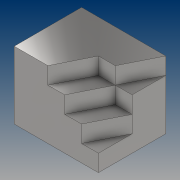
# Autodesk Inventor part: 23
Saved by Autodesk Inventor 2020.2 (Build 242310000, 310)
## iProperties
Created: 2020-09-17
Part Number: 23
Material: 鋼、碳鋼
Document SubType Name: Modeling
Designer: user
Density: 7.85 g/cm^3
Appearance: 半拋光
Mass: 549.5 g
Surface Area: 108.944 cm^2
Volume: 70 cm^3
Author: user
Autodesk Inventor part; units mm, degrees
ref_plane "YZ Plane" through (0, 0, 0) normal (1, 0, 0) x (0, 1, 0)
ref_plane "XZ Plane" through (0, 0, 0) normal (0, 1, 0) x (-1, 0, 0)
ref_plane "XY Plane" through (0, 0, 0) normal (0, 0, 1) x (1, 0, 0)
sketch "草圖1" plane through (0, 0, 0) normal (0, 1, 0) x (-1, 0, 0)
  line L0 (-25, 20) -> (25, 20)
  line L1 (25, 20) -> (25, -20)
  line L2 (25, -20) -> (-25, -20)
  line L3 (-25, -20) -> (-25, 20)
  line L4 (-25, 20) -> (25, -20) construction
  line L5 (25, 20) -> (-25, -20) construction
  point P0 (0, 0)
  dimension "d0" = 50
  dimension "d1" = 40
  constraints: 12 end point, 2 midpoint, 2 parallel, 1 horizontal, 1 perpendicular
  measures "d0" distance of L1.end L2.end
  measures "d1" distance of L0.end L1.end
extrude "擠出1" add sketch "草圖1" along normal blind 40
sketch "草圖2" plane through (0, 40, 0) normal (0, 1, 0) x (1, 0, 0)
  line L0 (-25, 20) -> (25, 20) projected
  line L1 (25, 20) -> (25, -20) projected
  line L2 (25, -20) -> (-25, -20) projected
  line L3 (-25, -20) -> (-25, 20) projected
  line L4 (15, -20) -> (25, 0)
  point P0 (0, 0)
  dimension "d4" = 10
  dimension "d5" = 20
  constraints: 2 end point, 1 midpoint, 1 point on line
  measures "d4" distance from line of L1 L4.start
  measures "d5" distance from line of L4.end L2
extrude "擠出2" cut sketch "草圖2" against normal blind 30 contours L1 L2 L4
sketch "草圖3" plane through (0, 40, 0) normal (0, 1, 0) x (1, 0, 0)
  line L0 (25, 0) -> (15, -20) projected
  line L1 (15, -20) -> (-25, -20) projected
  line L2 (-25, -20) -> (-25, 20) projected
  line L3 (-25, 20) -> (25, 20) projected
  line L4 (25, 20) -> (25, 0) projected
  line L5 (5, -20) -> (25, 20)
  line L6 (25, 0) -> (25, -20) projected
  point P0 (0, 0)
  dimension "d8" = 20
  constraints: 2 end point, 1 point on line
  measures "d8" distance from line of L6 L5.start
extrude "擠出3" cut sketch "草圖3" against normal blind 20 contours L0 L1 L5 L4
sketch "草圖4" plane through (0, 40, 0) normal (0, 1, 0) x (1, 0, 0)
  line L0 (25, 20) -> (5, -20) projected
  line L1 (5, -20) -> (-25, -20) projected
  line L2 (-25, -20) -> (-25, 20) projected
  line L3 (-25, 20) -> (25, 20) projected
  line L4 (-5, -20) -> (5, 0)
  line L5 (5, 0) -> (15, 0)
  line L6 (25, 0) -> (25, -20) projected
  point P0 (0, 0)
  dimension "d11" = 20
  dimension "d12" = 30
  dimension "d13" = 10
  constraints: 4 end point, 1 horizontal, 1 midpoint, 1 point on line
  measures "d11" distance between parallel lines of L1 L5
  measures "d12" distance from line of L6 L4.start
  measures "d13" distance of L4.end L5.end
extrude "擠出4" cut sketch "草圖4" against normal blind 10 contours L0 L1 L4 L5
sketch "草圖5" plane through (0, 20, 0) normal (0, 1, 0) x (1, 0, 0)
  line L0 (25, 20) -> (5, -20) projected
  line L1 (15, -20) -> (5, -20) projected
  line L2 (25, 0) -> (15, -20) projected
  line L3 (25, 20) -> (25, 0) projected
  line L4 (-25, 20) -> (25, 20) projected
  line L5 (-25, -20) -> (-25, 20) projected
  line L6 (5, -20) -> (-25, -20) projected
  line L7 (25, 0) -> (15, 0)
  line L8 (5, -20) -> (25, 20) projected
  point P0 (0, 0)
  constraints: 2 end point, 1 midpoint
extrude "擠出5" add sketch "草圖5" along normal blind 10 contours L3 L7 L0
